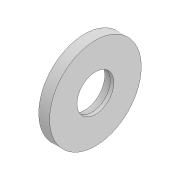
# Autodesk Inventor part: 200724 - Optotune adapter v1
Saved by Autodesk Inventor 2020.3 (Build 243373000, 373)
## iProperties
Created: 2020-07-24
Part Number: 200724 - Optotune adapter v1
Material: Generic
Document SubType Name: Modeling
Designer: Ralf
Density: 1 g/cm^3
Appearance: Default
Author: Ralf
Autodesk Inventor part; units mm, degrees
ref_plane "YZ Plane" through (0, 0, 0) normal (1, 0, 0) x (0, 1, 0)
ref_plane "XZ Plane" through (0, 0, 0) normal (0, 1, 0) x (-1, 0, 0)
ref_plane "XY Plane" through (0, 0, 0) normal (0, 0, 1) x (1, 0, 0)
sketch "Sketch1" plane through (0, 0, 0) normal (1, 0, 0) x (0, 1, 0)
  circle A0 centre (0, 0) radius 12.65
  dimension "d0" = 25.3
  constraints: 1 centre point, 1 coincident
  measures "d0" diameter of A0
extrude "Extrusion1" add sketch "Sketch1" along normal blind 3
sketch "Sketch2" plane through (3, 0, 0) normal (1, 0, 0) x (0, 0, -1)
  circle A0 centre (0, 0) radius 5.1
  dimension "d3" = 10.2
  constraints: 1 centre point, 1 coincident
  measures "d3" diameter of A0
extrude "Extrusion2" cut sketch "Sketch2" against normal blind 10
sketch "Sketch3" plane through (0, 0, 0) normal (-1, 0, 0) x (0, 0, 1)
  circle A0 centre (0, 0) radius 5.6
  circle A1 centre (0, 0) radius 5.1 projected
  line L0 (5.1, 0) -> (5.1, 2.313)
  line L1 (5.1, 0) -> (5.1, -2.313)
  dimension "d6" = 11.2
  constraints: 4 end point, 2 point on circle, 2 vertical, 1 centre point, 1 coincident, 1 horizontal alignment, 1 point on line, 1 other
  measures "d6" diameter of A0
extrude "Extrusion3" cut sketch "Sketch3" against normal blind 2 contours A1 | L0 L1 A0 picked at (-5.3273, 0.863)
body "Solid1"
